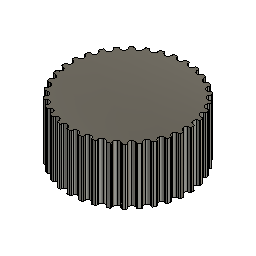
gear_34z (Autodesk Fusion 360 design; units mm, degrees)
Autodesk Fusion 360 part; units mm, degrees
sketch "Sketch1" plane through (0, 0, 0) normal (0, 0, 1) x (1, 0, 0) in component "gt2 pulley"
  circle A0 centre (0, 0) radius 10.8225 construction
  circle A1 centre (0, 0) radius 9.8185 construction
  line L0 (0, 0) -> (0, 10.8225) construction
  line L1 (0, 0) -> (0.9986, 10.7764) construction
  line L2 (0, 0) -> (1.4095, 10.7304) construction
  circle A2 centre (0, 0) radius 10.5685 construction
  arc A3 (0.3779, 10.4242) -> (0.4343, 10.1431) centre (1.3764, 10.4785) ccw
  circle A4 centre (0, 0) radius 10.4185 construction
  arc A5 (0.2313, 10.566) -> (0, 10.5685) centre (0, 0) ccw
  arc A6 (0.3779, 10.4242) -> (0.2313, 10.566) centre (0.2281, 10.416) ccw
  arc A7 (0.4343, 10.1431) -> (0.9059, 9.7767) centre (0.9571, 10.3293) ccw
  arc A8 (0, 10.5685) -> (-0.2313, 10.566) centre (0, 0) ccw
  arc A9 (-0.2313, 10.566) -> (-0.3779, 10.4242) centre (-0.2281, 10.416) ccw
  arc A10 (-0.4343, 10.1431) -> (-0.3779, 10.4242) centre (-1.3764, 10.4785) ccw
  arc A11 (-0.9057, 9.7767) -> (-0.4343, 10.1431) centre (-0.9571, 10.3293) ccw
  arc A12 (0.9059, 9.7767) -> (-0.9059, 9.7767) centre (0, 0) ccw
  point P0 (1.3764, 10.4785)
  point P1 (0, 10.5685)
  dimension "d18" = 21.6451
  dimension "d19" = 5.294
  dimension "d22" = 1.004
  dimension "d24" = 0.75
  dimension "d26" = 1
  dimension "d27" = 0.15
  dimension "d28" = 0.15
  dimension "d47" = 0.555
  dimension "d52" = 3.812
  constraint coincident A0.centre A1.centre
  constraint coincident A0 L0.end
  constraint vertical L0
  constraint coincident A0 L1.end
  constraint coincident A0 L2.end
  constraint concentric A1 A2
  constraint coincident A1 A7.end
  constraint coincident L1 A7.end
  constraint coincident A2 P0
  constraint coincident L2 P0
  constraint coincident P0 A3.centre
  constraint coincident A2 P1
  constraint coincident L0 P1
  constraint concentric A2 A4
  constraint coincident P1 A5.end
  constraint coincident A4 A6.centre
  constraint coincident A3.start A6.start
  constraint tangent A3 A6
  constraint tangent A3 A7
  constraint symmetric L0 A7.end A12.end
  constraint symmetric L0 A3.start A9.end
  constraint symmetric L0 A3.end A10.start
  constraint symmetric L0 A3 A10
  constraint symmetric L0 A5.start A8.end
  constraint symmetric L0 P1 A5.end
  constraint symmetric L0 A5 A8
  constraint symmetric L0 A6 A9
  constraint symmetric L0 A7 A11
  constraint coincident A1 A11.start
  constraint tangent A1 A7
  constraint coincident L1 A7.centre
  measures "d18" diameter of A0
  measures "d19" angle of L0 L1
  measures "d22" distance of A0 A1
  measures "d24" distance of A1 A2
  measures "d26" radius of A3
  measures "d27" distance of A2 A4
  measures "d28" radius of A6
  measures "d47" radius of A7
extrude "Extrude1" add sketch "Sketch1" along normal blind 10 makes body 1
pattern_circular "C-Pattern1" count 34 over 360 about axis through (0, 0, 1.75) along (0, 0, 1) of bodies 1 makes body 2 at (-2.4923, 9.497, 6.6667) makes body 3 at (-3.6405, 9.1187, 6.6667) makes body 4 at (-4.556, 8.6975, 3.3333) makes body 5 at (-6.6887, 7.1878, 6.6667) makes body 6 at (-7.3902, 6.4644, 3.3333) makes body 7 at (-8.8336, 4.2862, 6.6667) makes body 8 at (-9.2264, 3.3582, 3.3333) makes body 9 at (-9.6864, 1.6056, 3.3333) makes body 10 at (-9.6864, -1.6054, 6.6667) makes body 11 at (-9.4157, -2.7836, 6.6667) makes body 12 at (-9.0808, -3.7341, 3.3333) makes body 13 at (-8.24, -5.3391, 3.3333) makes body 14 at (-7.1187, -6.7623, 3.3333) makes body 15 at (-4.5562, -8.6974, 6.6667) makes body 16 at (-3.4528, -9.1914, 6.6667) makes body 17 at (-2.4925, -9.4969, 3.3333) makes body 18 at (-0.705, -9.7932, 3.3333) makes body 19 at (2.4923, -9.497, 6.6667) makes body 20 at (3.6405, -9.1187, 6.6667) makes body 21 at (4.556, -8.6975, 3.3333) makes body 22 at (6.6887, -7.1878, 6.6667) makes body 23 at (7.3902, -6.4644, 3.3333) makes body 24 at (8.4522, -4.9963, 3.3333) makes body 25 at (9.2264, -3.3582, 3.3333) makes body 26 at (9.6864, -1.6056, 3.3333) makes body 27 at (9.7669, 1.0061, 6.6667) makes body 28 at (9.6123, 2.0019, 3.3333) makes body 29 at (9.0808, 3.7341, 3.3333) makes body 30 at (8.24, 5.3391, 3.3333) makes body 31 at (6.54, 7.3234, 6.6667) makes body 32 at (5.7549, 7.9552, 3.3333) makes body 33 at (2.8805, 9.3865, 6.6667) makes body 34 at (2.4925, 9.4969, 3.3333)
sketch "Sketch2" plane through (0, 0, 10) normal (0, 0, 1) x (-1, 0, 0)
  arc A0 (-5.8089, -8.6639) -> (-5.7589, -8.8616) centre (-5.6773, -8.7358) ccw
  arc A1 (-5.7589, -8.8616) -> (-5.3656, -9.1052) centre (0, 0) ccw
  arc A2 (-5.3656, -9.1052) -> (-5.1664, -9.0617) centre (-5.2894, -8.976) ccw
  arc A3 (-4.9704, -8.8525) -> (-5.1664, -9.0617) centre (-4.346, -9.6336) ccw
  arc A4 (-4.3767, -8.7891) -> (-4.9704, -8.8525) centre (-4.6239, -9.286) ccw
  arc A5 (-5.917, -7.8354) -> (-4.3767, -8.7891) centre (0, 0) ccw
  arc A6 (-5.7089, -8.3953) -> (-5.917, -7.8354) centre (-6.2515, -8.2783) ccw
  arc A7 (-5.8089, -8.6639) -> (-5.7089, -8.3953) centre (-6.6865, -8.1845) ccw
  circle A8 centre (0, 0) radius 9.8185
  constraint coincident A1.centre A5.centre
extrude "Extrude2" add sketch "Sketch2" against normal blind 10 contours A5 A8 bodies 1 2 3 4 5 6 7 8 9 10 11 12 13 14 15 16 17 18 19 20 21 22 23 24 25 26 27 28 29 30 31 32 33 34
extrude "Extrude4" [suppressed] in component "gt2 pulley"
pattern_circular "C-Pattern7" [suppressed] in component "gt2 pulley"
extrude "Extrude3" [suppressed] in component "gt2 pulley"
pattern_circular "C-Pattern6" [suppressed] in component "gt2 pulley"
extrude "Extrude2'" [suppressed] in component "gt2 pulley"
pattern_circular "C-Pattern5" [suppressed] in component "gt2 pulley"
extrude "Extrude1'" [suppressed] in component "gt2 pulley"
pattern_circular "C-Pattern4" [suppressed] in component "gt2 pulley"
pattern_circular "C-Pattern3" [suppressed] in component "gt2 pulley"
pattern_circular "C-Pattern2" [suppressed] in component "gt2 pulley"
pattern_circular "C-Pattern1'" [suppressed] in component "gt2 pulley"
copy_body "Body->Comp1" [suppressed] in component "Component"
copy_body "Body->Comp2" [suppressed] in component "Component'"
copy_body "Body->Comp3" [suppressed] in component "Component''"
copy_body "Body->Comp4" [suppressed] in component "Component'''"
copy_body "Body->Comp5" [suppressed] in component "Component''''"
copy_body "Body->Comp6" [suppressed] in component "Component'''''"
copy_body "Body->Comp7" [suppressed] in component "Component''''''"
copy_body "Body->Comp8" [suppressed] in component "Component'''''''"
copy_body "Body->Comp9" [suppressed] in component "Component''''''''"
copy_body "Body->Comp10" [suppressed] in component "Component'''''''''"
copy_body "Body->Comp11" [suppressed] in component "Component''''''''''"
copy_body "Body->Comp12" [suppressed] in component "Component'''''''''''"
copy_body "Body->Comp13" [suppressed] in component "Component''''''''''''"
copy_body "Body->Comp14" [suppressed] in component "Component'''''''''''''"
copy_body "Body->Comp15" [suppressed] in component "Component''''''''''''''"
copy_body "Body->Comp16" [suppressed] in component "Component'''''''''''''''"
copy_body "Body->Comp17" [suppressed] in component "Component''''''''''''''''"
copy_body "Body->Comp18" [suppressed] in component "Component'''''''''''''''''"
copy_body "Body->Comp19" [suppressed] in component "Component''''''''''''''''''"
copy_body "Body->Comp20" [suppressed] in component "Component'''''''''''''''''''"
component "gt2 pulley" placed x (1, 0, 0) y (0, 1, 0) z (0, 0, 1) at (0, 0, 0)
equation "NumTeeth = 34" comment "min 20"
equation "ToothPitch = 2 mm"
equation "PullyDia = NumTeeth * ToothPitch / PI"
equation "ToothAng = ( ( 360 / NumTeeth ) * 1 deg )"
equation "TransOffsetAngle = ToothAng * 0.2"
equation "Sholulder_Radius = 0.15 mm"
equation "Root_Radius = 0.555 mm"
equation "TransRadius = 1 mm"
equation "ToolHeight = 0.75 mm"
equation "PLD = 0.254 mm"
equation "d18 = PullyDia"
equation "d19 = ToothAng / 2"
equation "d22 = PLD + ToolHeight"
equation "d24 = ToolHeight"
equation "d26 = TransRadius"
equation "d27 = Sholulder_Radius"
equation "d31 = NumTeeth"
equation "d33 = NumTeeth"
equation "d35 = NumTeeth"
equation "d37 = NumTeeth"
equation "d41 = NumTeeth"
equation "d45 = NumTeeth"
equation "d47 = Root_Radius"
equation "d50 = NumTeeth"
